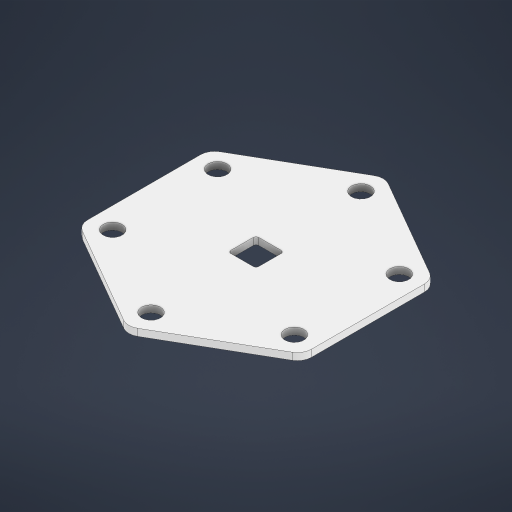
# Autodesk Inventor part: Flex wheel mount polycarb
Saved by Autodesk Inventor 2023 (Build 270158000, 158)
## iProperties
Created: 2023-03-22
Part Number: Flex wheel mount polycarb
Material: Polycarbonate, Clear
Document SubType Name: Modeling
Designer: Main Account
Density: 1.2 g/cm^3
Appearance: White
Author: Main Account
Autodesk Inventor part; units mm, degrees
ref_plane "YZ Plane" through (0, 0, 0) normal (1, 0, 0) x (0, 1, 0)
ref_plane "XZ Plane" through (0, 0, 0) normal (0, 1, 0) x (-1, 0, 0)
ref_plane "XY Plane" through (0, 0, 0) normal (0, 0, 1) x (1, 0, 0)
sketch "Sketch1" plane through (0, 0, 0) normal (0, 1, 0) x (-1, 0, 0)
  circle A0 centre (-20.6222, -11.9063) radius 2.1526
  line L0 (1.5875, 28.4129) -> (23.8125, 15.5812)
  line L1 (25.4, 12.8316) -> (25.4, -12.8316)
  line L2 (23.8125, -15.5812) -> (1.5875, -28.4129)
  line L3 (-1.5875, -28.4129) -> (-23.8125, -15.5812)
  line L4 (-25.4, -12.8316) -> (-25.4, 12.8316)
  line L5 (-23.8125, 15.5812) -> (-1.5875, 28.4129)
  arc A1 (-23.8125, 15.5812) -> (-25.4, 12.8316) centre (-22.225, 12.8316) ccw
  arc A2 (1.5875, 28.4129) -> (-1.5875, 28.4129) centre (0, 25.6632) ccw
  arc A3 (25.4, 12.8316) -> (23.8125, 15.5812) centre (22.225, 12.8316) ccw
  arc A4 (23.8125, -15.5812) -> (25.4, -12.8316) centre (22.225, -12.8316) ccw
  arc A5 (-25.4, -12.8316) -> (-23.8125, -15.5812) centre (-22.225, -12.8316) ccw
  arc A6 (-1.5875, -28.4129) -> (1.5875, -28.4129) centre (0, -25.6632) ccw
  line L6 (2.5146, -3.175) -> (-2.5146, -3.175)
  line L7 (-3.175, -2.5146) -> (-3.175, 2.5146)
  line L8 (-2.5146, 3.175) -> (2.5146, 3.175)
  line L9 (3.175, 2.5146) -> (3.175, -2.5146)
  line L10 (3.175, -3.175) -> (-3.175, 3.175) construction
  line L11 (-3.175, -3.175) -> (3.175, 3.175) construction
  arc A7 (-2.5146, 3.175) -> (-3.175, 2.5146) centre (-2.5146, 2.5146) ccw
  arc A8 (3.175, 2.5146) -> (2.5146, 3.175) centre (2.5146, 2.5146) ccw
  arc A9 (-3.175, -2.5146) -> (-2.5146, -3.175) centre (-2.5146, -2.5146) ccw
  arc A10 (2.5146, -3.175) -> (3.175, -2.5146) centre (2.5146, -2.5146) ccw
  circle A11 centre (-20.6222, -11.9063) radius 2.1526
  circle A12 centre (0, -23.8125) radius 2.1526
  circle A13 centre (20.6222, -11.9062) radius 2.1526
  circle A14 centre (0, 23.8125) radius 2.1526
  circle A15 centre (20.6222, 11.9063) radius 2.1526
  circle A16 centre (-20.6222, 11.9062) radius 2.1526
  point P0 (0, 0)
  point P1 (0, 29.3294)
  point P2 (25.4, 14.6647)
  point P3 (25.4, -14.6647)
  point P4 (0, -29.3294)
  point P5 (-25.4, -14.6647)
  point P6 (-25.4, 14.6647)
  point P7 (0, 0)
  dimension "d0" = 3.175
  dimension "d1" = 3.175
  dimension "d2" = 6.35
  dimension "d3" = 6.35
  constraints: 24 end point, 20 point on circle, 20 tangent, 17 centre point, 13 coincident, 12 point on line, 5 equal radius, 2 midpoint, 2 parallel, 1 horizontal, 1 perpendicular
  measures "d0" radius of A1
  measures "d1" radius of A5
  measures "d2" distance of L10.end L11.end
  measures "d3" distance of L11.start L10.end
extrude "Extrusion1" add sketch "Sketch1" along normal blind 1.5875
body "Solid1"
